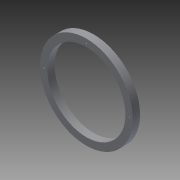
# Autodesk Inventor part: TSOP Ring
Saved by Autodesk Inventor 2015 (Build 190159000, 159)
## iProperties
Created: 2016-08-09
Part Number: TSOP Ring
Material: Generic
Document SubType Name: Modeling
Designer: James Yelland
Density: 1 g/cm^3
Appearance: Default
Author: James Yelland
Autodesk Inventor part; units mm, degrees
ref_plane "YZ Plane" through (0, 0, 0) normal (1, 0, 0) x (0, 1, 0)
ref_plane "XZ Plane" through (0, 0, 0) normal (0, 1, 0) x (-1, 0, 0)
ref_plane "XY Plane" through (0, 0, 0) normal (0, 0, 1) x (1, 0, 0)
sketch "Sketch1" plane through (0, 0, 0) normal (0, 1, 0) x (-1, 0, 0)
  circle A0 centre (0, 0) radius 95
  circle A1 centre (0, 0) radius 80
  circle A2 centre (0, 87.5) radius 1.6
  circle A3 centre (-87.5, 0) radius 1.6
  circle A4 centre (87.5, 0) radius 1.6
  circle A5 centre (0, 0) radius 105
  line L0 (0, -105) -> (0, -85)
  line L1 (0, -85) -> (-61.6441, -85)
  line L2 (0, -85) -> (61.6441, -85)
  dimension "d0" = 190
  dimension "d1" = 160
  dimension "d4" = 3.2
  dimension "d5" = 3.2
  dimension "d6" = 3.2
  dimension "d7" = 210
  dimension "d8" = 20
  constraints: 6 centre point, 6 end point, 3 coincident, 3 point on circle, 1 perpendicular, 1 point on line, 1 vertical
  measures "d0" diameter of A0
  measures "d1" diameter of A1
  measures "d4" diameter of A2
  measures "d5" diameter of A3
  measures "d6" diameter of A4
  measures "d7" diameter of A5
  measures "d8" distance of L0.start L0.end
extrude "Extrusion1" add sketch "Sketch1" along normal blind 15 contours A0 L2 L1 | L1 L0 A0 | A0 L0 L2
body "Solid1"
